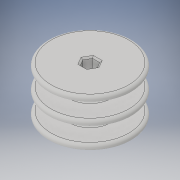
# Autodesk Inventor part: spool
Saved by Autodesk Inventor 2019.3 (Build 233278000, 278)
## iProperties
Created: 2019-02-25
Part Number: spool
Material: Generic
Document SubType Name: Modeling
Designer: steele
Density: 1 g/cm^3
Appearance: Default
Author: steele
Autodesk Inventor part; units mm, degrees
ref_plane "YZ Plane" through (0, 0, 0) normal (1, 0, 0) x (0, 1, 0)
ref_plane "XZ Plane" through (0, 0, 0) normal (0, 1, 0) x (-1, 0, 0)
ref_plane "XY Plane" through (0, 0, 0) normal (0, 0, 1) x (1, 0, 0)
sketch "Sketch1" plane through (0, 0, 0) normal (1, 0, 0) x (0, 1, 0)
  line L0 (0, 0) -> (0, -41.275)
  line L1 (3.175, -44.45) -> (3.175, -44.45)
  line L2 (6.35, -41.275) -> (6.35, -22.225)
  line L3 (9.525, -19.05) -> (19.05, -19.05)
  line L4 (22.225, -22.225) -> (22.225, -41.275)
  line L5 (25.4, -44.45) -> (25.4, -44.45)
  line L6 (28.575, -41.275) -> (28.575, -22.225)
  line L7 (31.75, -19.05) -> (41.275, -19.05)
  line L8 (44.45, -22.225) -> (44.45, -41.275)
  line L9 (47.625, -44.45) -> (47.625, -44.45)
  line L10 (50.8, -41.275) -> (50.8, 0)
  line L11 (0, 0) -> (50.8, 0)
  arc A0 (47.625, -44.45) -> (50.8, -41.275) centre (47.625, -41.275) ccw
  arc A1 (44.45, -41.275) -> (47.625, -44.45) centre (47.625, -41.275) ccw
  arc A2 (25.4, -44.45) -> (28.575, -41.275) centre (25.4, -41.275) ccw
  arc A3 (22.225, -41.275) -> (25.4, -44.45) centre (25.4, -41.275) ccw
  arc A4 (3.175, -44.45) -> (6.35, -41.275) centre (3.175, -41.275) ccw
  arc A5 (0, -41.275) -> (3.175, -44.45) centre (3.175, -41.275) ccw
  arc A6 (44.45, -22.225) -> (41.275, -19.05) centre (41.275, -22.225) ccw
  arc A7 (31.75, -19.05) -> (28.575, -22.225) centre (31.75, -22.225) ccw
  arc A8 (22.225, -22.225) -> (19.05, -19.05) centre (19.05, -22.225) ccw
  arc A9 (9.525, -19.05) -> (6.35, -22.225) centre (9.525, -22.225) ccw
  point P0 (44.45, -44.45)
  point P1 (50.8, -44.45)
  dimension "d0" = 50.8
  dimension "d1" = 6.35
  dimension "d2" = 19.05
  dimension "d3" = 44.45
  dimension "d4" = 3.175
  dimension "d5" = 3.175
  constraints: 24 end point, 20 point on circle, 20 tangent, 10 centre point, 8 equal radius, 6 perpendicular, 6 point on line, 5 collinear, 1 horizontal, 1 parallel, 1 vertical
  measures "d0" distance between parallel lines of L10 L0
  measures "d1" distance of point (44.45, -44.45) point (50.8, -44.45)
  measures "d2" distance between parallel lines of L3 L11
  measures "d3" distance between parallel lines of L1 L11
  measures "d4" radius of A0
  measures "d5" radius of A6
revolve "Revolution1" add sketch "Sketch1" angle 360 about axis through (0, 0, 0) along (0, 1, 0)
sketch "Sketch2" plane through (0, 50.8, 0) normal (0, 1, 0) x (1, 0, 0)
  line L0 (7.6623, 0) -> (3.8312, -6.6357)
  line L1 (3.8312, -6.6357) -> (-3.8312, -6.6357)
  line L2 (-3.8312, -6.6357) -> (-7.6623, 0)
  line L3 (-7.6623, 0) -> (-3.8312, 6.6357)
  line L4 (-3.8312, 6.6357) -> (3.8312, 6.6358)
  line L5 (3.8312, 6.6358) -> (7.6623, 0)
  point P0 (0, 0)
  point P1 (0, 0)
  dimension "d8" = 13.2715
  constraints: 12 end point, 1 coincident, 1 horizontal, 13 other
  measures "d8" distance between parallel lines of L1 L4
extrude "Extrusion1" cut sketch "Sketch2" against normal through all
sketch "Sketch4" plane through (0, 0, 0) normal (1, 0, 0) x (0, 1, 0)
  circle A0 centre (36.5125, 8.3858) radius 1.75
  circle A1 centre (14.2875, 8.3858) radius 1.75
  line L0 (6.35, 41.275) -> (6.35, -41.275) projected
  line L1 (44.45, 41.275) -> (44.45, -41.275) projected
  line L2 (50.8, 0) -> (0, 0) projected
  dimension "d17" = 7.9375
  dimension "d18" = 7.9375
  dimension "d19" = 3.5
  dimension "d20" = 8.3857
  dimension "d21" = 8.3857
  constraints: 2 centre point, 1 equal radius
  measures "d17" distance from line of A1.centre L0
  measures "d18" distance from line of A0.centre L1
  measures "d19" diameter of A0
  measures "d20" distance from line of A1.centre L2
  measures "d21" distance from line of A0.centre L2
extrude "Extrusion3" cut sketch "Sketch4" along normal through all both and the other way through all
chamfer "Chamfer2" distance 1.5875 angle 45 12 edges at (-5.7467, 50.8, -3.3179) (-5.7467, 50.8, 3.3179) (0, 50.8, 6.6357) (5.7467, 50.8, 3.3179) (0, 50.8, -6.6358) (0, 0, 6.6357) (5.7467, 0, 3.3179) (5.7467, 0, -3.3179) (0, 0, -6.6358) (-5.7467, 0, -3.3179) (-5.7467, 0, 3.3179) (5.7467, 50.8, -3.3179)
equation "\"d0\" = spoolHeight"
equation "\"d1\" = supportChannels"
equation "\"d2\" = spoolInteriroRadius"
equation "\"d3\" = spoolExteriorRadius"
equation "\"d4\" = spoolFiletRadius"
equation "\"d5\" = spoolFiletRadius"
equation "\"d8\" = hexDiameter"
equation "\"d17\" = holeCenter"
equation "\"d18\" = holeCenter"
equation "\"d19\" = holeForString"
equation "\"d20\" = stringHoleCenterFromHexShaft"
equation "\"d21\" = stringHoleCenterFromHexShaft"
equation "\"d27\" = hexHoleChamfer"
equation "\"holeForString\" = stringDiameter + clearanceForString"
equation "\"stringDiameter\" = 3"
equation "\"clearanceForString\" = 0.5"
equation "\"spoolHeight\" = 50.8"
equation "\"hexShaftDiameter\" = 12.7"
equation "\"clearanceForHexShaft\" = 0.5715"
equation "\"hexDiameter\" = hexShaftDiameter + clearanceForHexShaft"
equation "\"supportChannels\" = 6.35"
equation "\"spoolInteriorDiameter\" = 38.1"
equation "\"spoolInteriroRadius\" = 0.5 * spoolInteriorDiameter"
equation "\"spoolExteriorDiameter\" = 88.9"
equation "\"spoolExteriorRadius\" = 0.5 * spoolExteriorDiameter"
equation "\"spoolFiletRadius\" = 0.5 * supportChannels"
equation "\"holeCenter\" = 0.25 * spoolHeight - 0.75 * supportChannels"
equation "\"hexHoleChamfer\" = 1.5875"
equation "\"stringHoleCenterFromHexShaft\" = 0.5 * hexDiameter + 0.5 * holeForString"
body "Solid1"
